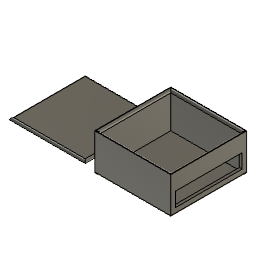
relais_box_v1 (Autodesk Fusion 360 design; units mm, degrees)
part number: 2026-08-18-10-48-03-888
Autodesk Fusion 360 part; units mm, degrees
sketch "Sketch1" plane through (0, 0, 0) normal (0, 0, 1) x (1, 0, 0)
  line L0 (0, 0) -> (80, 0)
  line L1 (80, 0) -> (80, 80)
  line L2 (80, 80) -> (0, 80)
  line L3 (0, 80) -> (0, 0)
extrude "Extrude1" add sketch "Sketch1" along normal blind 40 makes body 1
shell "Shell1" thickness 3 removed faces 1 at (26.6667, 53.3333, 40) on bodies 1
ref_plane "WorkPlane1" through (0, 0, 47) normal (0, 0, 1) x (1, 0, 0)
sketch "Sketch2" plane through (0, 0, 47) normal (0, 0, 1) x (1, 0, 0)
  line L0 (0, 0) -> (80, 0)
  line L1 (80, 0) -> (80, 80)
  line L2 (80, 80) -> (0, 80)
  line L3 (0, 80) -> (0, 0)
extrude "Extrude2" add sketch "Sketch2" against normal blind 2 separate body makes body 2
ref_plane "WorkPlane2" through (0, 0, 40) normal (0, 0, 1) x (1, 0, 0)
sketch "Sketch3" plane through (0, 0, 40) normal (0, 0, 1) x (1, 0, 0)
  line L0 (3.5, 3.5) -> (76.5, 3.5)
  line L1 (76.5, 3.5) -> (76.5, 76.5)
  line L2 (76.5, 76.5) -> (3.5, 76.5)
  line L3 (3.5, 76.5) -> (3.5, 3.5)
extrude "Extrude3" add sketch "Sketch3" along normal blind 5 bodies 2
fillet "Fillet1" radius 2.5 8 edges at (40, 77, 40) (77, 40, 40) (40, 3, 40) (3, 40, 40) (40, 80, 0) (80, 40, 0) (40, 0, 0) (0, 40, 0) on bodies 1
fillet "Fillet2" radius 2.5 8 edges at (40, 76.5, 40) (76.5, 40, 40) (40, 3.5, 40) (3.5, 40, 40) (40, 0, 47) (80, 40, 47) (40, 80, 47) (0, 40, 47) on bodies 2
move_body "Move1" bodies 2 to x (1, 0, 0) y (0, 1, 0) z (0, 0, 1) at (-90, 0, -40)
sketch "Sketch4" plane through (80, 0, 0) normal (1, 0, 0) x (0, 1, 0)
  line L0 (0, 2.5) -> (80, 2.5)
  line L1 (80, 2.5) -> (80, 40)
  line L2 (80, 40) -> (0, 40)
  line L3 (0, 40) -> (0, 2.5)
  line L4 (5, 3) -> (75, 3)
  line L5 (75, 3) -> (75, 18)
  line L6 (75, 18) -> (5, 18)
  line L7 (5, 18) -> (5, 3)
extrude "Extrude4" cut sketch "Sketch4" along normal blind 3 bodies 1
sketch "Sketch5" plane through (80, 0, 0) normal (1, 0, 0) x (0, 1, 0)
  line L0 (0, 2.5) -> (80, 2.5)
  line L1 (80, 2.5) -> (80, 40)
  line L2 (80, 40) -> (0, 40)
  line L3 (0, 40) -> (0, 2.5)
  line L4 (5, 22.5) -> (75, 22.5)
  line L5 (75, 22.5) -> (75, 7.5)
  line L6 (75, 7.5) -> (5, 7.5)
  line L7 (5, 7.5) -> (5, 22.5)
  dimension "d18" = 70
  dimension "d19" = 15
  dimension "d20" = 5
  dimension "d21" = 5
  constraint horizontal L4
  constraint vertical L5
  constraint horizontal L6
  constraint vertical L7
  measures "d18" distance of L4.start L4.end
  measures "d19" distance of L4.start L6.end
  measures "d20" distance of L3 L7
  measures "d21" distance of L0 L6
extrude "Extrude5" cut sketch "Sketch5" against normal blind 10 contours L4 L5 L6 L7 bodies 1
named bodies: "Box", "Lid"
